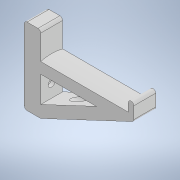
# Autodesk Inventor part: Spool Holder
Saved by Autodesk Inventor 2022 (Build 260153000, 153)
## iProperties
Created: 2022-03-03
Part Number: Spool Holder
Material: Generic
Document SubType Name: Modeling
Designer: Nick
Density: 1 g/cm^3
Appearance: Default
Author: Nick
Autodesk Inventor part; units mm, degrees
ref_plane "YZ Plane" through (0, 0, 0) normal (1, 0, 0) x (0, 1, 0)
ref_plane "XZ Plane" through (0, 0, 0) normal (0, 1, 0) x (-1, 0, 0)
ref_plane "XY Plane" through (0, 0, 0) normal (0, 0, 1) x (1, 0, 0)
sketch "Sketch1" plane through (0, 0, 0) normal (0, 0, 1) x (1, 0, 0)
  line L0 (0, 0) -> (0, 70)
  line L1 (0, 70) -> (15, 70)
  line L2 (15, 70) -> (15, 45)
  line L3 (15, 45) -> (95, 45)
  line L4 (95, 45) -> (95, 55)
  line L5 (95, 55) -> (100, 55)
  line L6 (100, 55) -> (100, 40)
  line L7 (100, 40) -> (15, 0)
  line L8 (15, 0) -> (0, 0)
  line L9 (100, 40) -> (95, 45) construction
  line L10 (15, 35) -> (65.8896, 35)
  line L11 (65.8896, 35) -> (15, 11.0519)
  line L12 (15, 11.0519) -> (15, 35)
  dimension "d0" = 5
  dimension "d1" = 80
  dimension "d2" = 70
  dimension "d3" = 25
  dimension "d4" = 15
  dimension "d5" = 15
  dimension "d6" = 10
  dimension "d7" = 135
  dimension "d8" = 10
  dimension "d9" = 10
  dimension "d10" = 15
  constraints: 26 end point, 3 horizontal, 3 parallel, 3 vertical, 2 perpendicular
  measures "d0" distance of L4.end L5.end
  measures "d1" distance of L2.end L3.end
  measures "d2" distance of L0.start L0.end
  measures "d3" distance of L1.end L2.end
  measures "d4" distance of L7.end L0.start
  measures "d5" distance of L0.end L1.end
  measures "d6" distance of L3.end L4.end
  measures "d7" angle of L4 L9
  measures "d8" distance between parallel lines of L3 L10
  measures "d9" distance between parallel lines of L7 L11
  measures "d10" distance between parallel lines of L0 L12
extrude "Extrusion1" add sketch "Sketch1" along normal blind 20
sketch "Sketch2" plane through (15, 11.0519, 0) normal (1, 0, 0) x (0, 0, -1)
  line L0 (0, 0) -> (0, 23.9481) projected
  line L1 (0, 23.9481) -> (-20, 23.9481) projected
  line L2 (-20, 0) -> (-20, 23.9481) projected
  line L3 (0, 0) -> (-20, 0) projected
  circle A0 centre (-10, 11.974) radius 4
  line L4 (0, 23.9481) -> (-20, 23.9481) construction
  line L5 (-10, 23.9481) -> (-10, 0) construction
  point P0 (0, -11.0519)
  dimension "d14" = 8
  constraints: 3 midpoint, 2 end point, 1 centre point
  measures "d14" diameter of A0
extrude "Extrusion2" cut sketch "Sketch2" along normal blind 71.75 contours A0
hole "Hole1" at (15, 23.026, 10) direction (-1, 0, 0) diameter 3.4036 end through all counterbore diameter 6.5024 counterbore depth 3.4036 clearance for "Socket Head Cap Screw ISO 4762" size "M3" standard "ISO"
sketch "Sketch3" plane through (15, 45, 0) normal (1, 0, 0) x (0, 0, -1)
  line L0 (0, 0) -> (0, 25) projected
  line L1 (0, 25) -> (-20, 25) projected
  line L2 (-20, 0) -> (-20, 25) projected
  line L3 (0, 0) -> (-20, 0) projected
  circle A0 centre (-10, -36.7642) radius 38.1
  point P0 (0, -45)
  dimension "d28" = 76.2
  constraints: 2 point on circle, 1 centre point
  measures "d28" diameter of A0
extrude "Extrusion3" add sketch "Sketch3" along normal up to surface (80 mm away) contours L3 A0 picked at (-11.1228, 0.3955)
fillet "Fillet1" radius 2.5 7 edges at (15, 70, 10) (0, 70, 10) (95, 55, 10) (100, 55, 10) (0, 0, 10) (15, 0, 10) (100, 40, 10)
equation "\"d4\" = d5"
equation "\"d10\" = d5"
equation "\"d14\" = d13"
equation "\"d13\" = 8"
body "Solid1"
